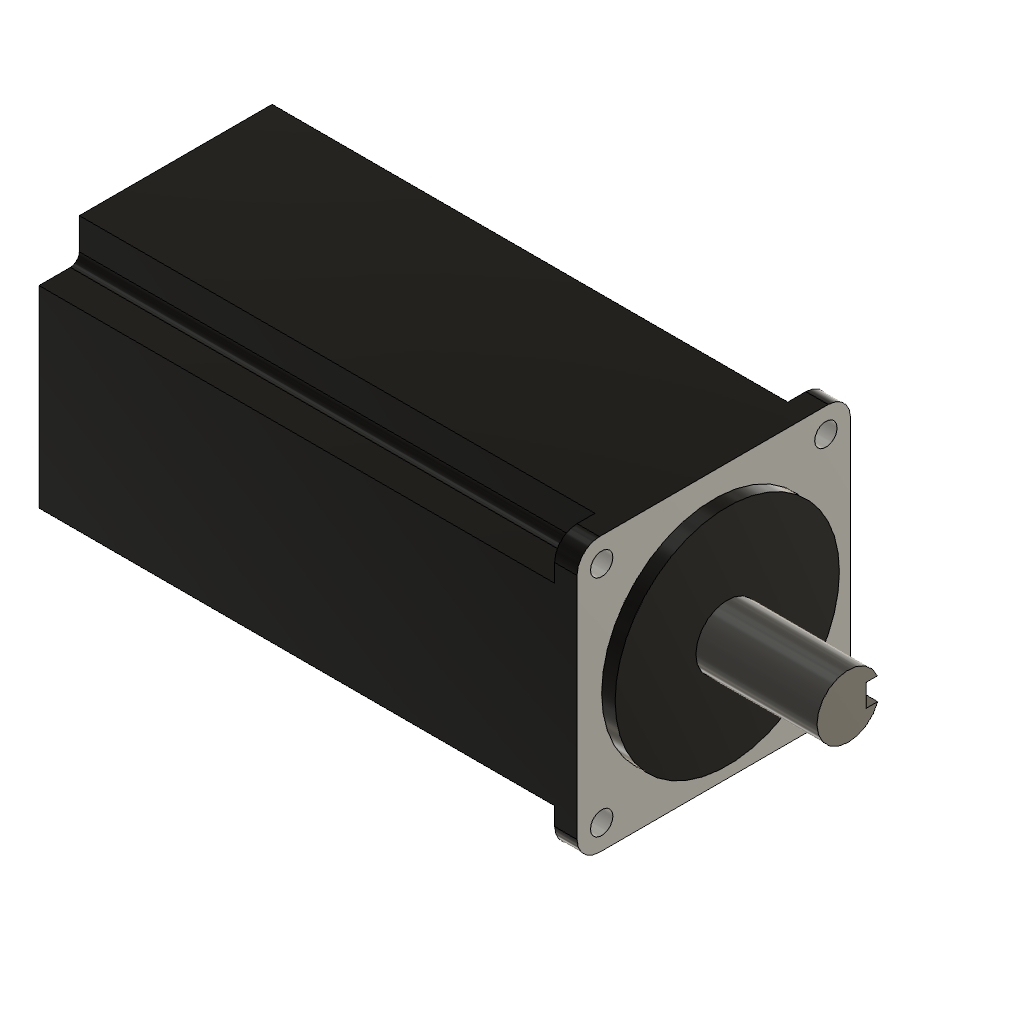
RobotRKO-dobrane elementy (Autodesk Fusion 360 archive; units mm, degrees)
design "NEMA24 60BL120"
part number: 2026-10-05-21-43-38-421
Autodesk Fusion 360 part; units mm, degrees
note: some values were not read from the file. Chosen so that the rebuilt part matches the saved one: a direction. Set by a fixed rule: which sketch regions a step uses.
sketch "Szkic1" plane through (0, 0, 0) normal (1, 0, 0) x (0, 1, 0)
  line L0 (30.5, 30.5) -> (-30.5, 30.5)
  line L1 (-30.5, 30.5) -> (-30.5, -30.5)
  line L2 (-30.5, -30.5) -> (30.5, -30.5)
  line L3 (30.5, -30.5) -> (30.5, 30.5)
  line L4 (30.5, 30.5) -> (-30.5, -30.5) construction
  line L5 (-30.5, 30.5) -> (30.5, -30.5) construction
  dimension "d1" = 61
  dimension "d2" = 61
  constraint horizontal L0
  constraint perpendicular L0 L1
  constraint parallel L0 L2
  constraint parallel L1 L3
  constraint coincident L4 origin
  constraint coincident L5 origin
  measures "d1" distance of L0.start L2.end
  measures "d2" distance of L1.end L2.end
extrude "Wyciągnięcie proste1" add sketch "Szkic1" along normal blind 120
sketch "Szkic2" plane through (120, 0, 0) normal (1, 0, 0) x (0, 1, 0)
  line L0 (30.5, -30.5) -> (30.5, 30.5)
  line L1 (30.5, 30.5) -> (-30.5, 30.5)
  line L2 (-30.5, 30.5) -> (-30.5, -30.5)
  line L3 (-30.5, -30.5) -> (30.5, -30.5)
  circle A0 centre (0, 0) radius 25
  dimension "d5" = 50
  constraint coincident A0.centre origin
  measures "d5" diameter of A0
extrude "Wyciągnięcie proste2" add sketch "Szkic2" along normal blind 3 contours A0
sketch "Szkic3" plane through (123, 0, 0) normal (1, 0, 0) x (0, 1, 0)
  circle A0 centre (0, 0) radius 25
  circle A1 centre (0, 0) radius 7
  dimension "d8" = 14
  constraint concentric A0 A1
  measures "d8" diameter of A1
extrude "Wyciągnięcie proste3" add sketch "Szkic3" along normal blind 27 contours A1
sketch "Szkic4" plane through (150, 0, 0) normal (1, 0, 0) x (0, 1, 0)
  circle A0 centre (0, 0) radius 7
  line L0 (4, -2.4) -> (4, 2.6)
  line L1 (4, 2.6) -> (6.4992, 2.6)
  line L2 (4, -2.4) -> (6.5757, -2.4)
  point P0 (4, 0.1)
  dimension "d11" = 5
  dimension "d12" = 4
  constraint midpoint L0 P0
  constraint vertical L0
  constraint coincident A0 L1.end
  constraint perpendicular L0 L1
  constraint coincident A0 L2.end
  constraint perpendicular L0 L2
  measures "d11" distance of L0.start L0.end
  measures "d12" distance of A0.centre L0
extrude "Wyciągnięcie proste4" cut sketch "Szkic4" against normal blind 25 contours A0 L0 L1 L2 picked at (5, 0.0667)
sketch "Szkic6" plane through (120, 0, 0) normal (1, 0, 0) x (0, 1, 0)
  circle A0 centre (0, 0) radius 25
  line L0 (30.5, -30.5) -> (30.5, 30.5)
  line L1 (30.5, 30.5) -> (-30.5, 30.5)
  line L2 (-30.5, 30.5) -> (-30.5, -30.5)
  line L3 (-30.5, -30.5) -> (30.5, -30.5)
  line L4 (25, -25) -> (-25, -25) construction
  line L5 (-25, -25) -> (-25, 25) construction
  line L6 (-25, 25) -> (25, 25) construction
  line L7 (25, 25) -> (25, -25) construction
  line L8 (25, -25) -> (-25, 25) construction
  line L9 (-25, -25) -> (25, 25) construction
  circle A1 centre (-25, 25) radius 2.5
  circle A2 centre (25, 25) radius 2.5
  circle A3 centre (-25, -25) radius 2.5
  circle A4 centre (25, -25) radius 2.5
  dimension "d15" = 50
  dimension "d16" = 50
  dimension "d17" = 5
  dimension "d20" = 50
  dimension "d21" = -50
  constraint horizontal L4
  constraint perpendicular L4 L5
  constraint parallel L4 L6
  constraint parallel L5 L7
  constraint coincident L8 A0.centre
  constraint coincident L9 A0.centre
  constraint coincident A0.centre origin
  constraint coincident L5.end L6.start
  measures "d15" distance of L4.start L6.end
  measures "d16" distance of L5.end L6.end
  measures "d17" diameter of A1
extrude "Wyciągnięcie proste5" cut sketch "Szkic6" against normal blind 120 contours A1 | A2 | A3 | A4
ref_plane "Płaszczyzna konstrukcyjna1" through (110, 0, 0) normal (1, 0, 0) x (0, 0, -1)
sketch "Szkic7" plane through (110, 0, 0) normal (1, 0, 0) x (0, 1, 0)
  line L0 (30.5, 30.5) -> (21.5, 30.5)
  line L1 (21.5, 30.5) -> (21.5, 23.5)
  line L2 (23.5, 21.5) -> (30.5, 21.5)
  line L3 (30.5, 21.5) -> (30.5, 30.5)
  arc A0 (21.5, 23.5) -> (23.5, 21.5) centre (23.5, 23.5) ccw
  line L4 (-30.5, 30.5) -> (-21.5, 30.5)
  line L5 (-21.5, 30.5) -> (-21.5, 23.5)
  line L6 (-23.5, 21.5) -> (-30.5, 21.5)
  line L7 (-30.5, 21.5) -> (-30.5, 30.5)
  arc A1 (-23.5, 21.5) -> (-21.5, 23.5) centre (-23.5, 23.5) ccw
  line L8 (-30.5, -30.5) -> (-21.5, -30.5)
  line L9 (-21.5, -30.5) -> (-21.5, -23.5)
  line L10 (-23.5, -21.5) -> (-30.5, -21.5)
  line L11 (-30.5, -21.5) -> (-30.5, -30.5)
  arc A2 (-21.5, -23.5) -> (-23.5, -21.5) centre (-23.5, -23.5) ccw
  line L12 (30.5, -30.5) -> (21.5, -30.5)
  line L13 (21.5, -30.5) -> (21.5, -23.5)
  line L14 (23.5, -21.5) -> (30.5, -21.5)
  line L15 (30.5, -21.5) -> (30.5, -30.5)
  arc A3 (23.5, -21.5) -> (21.5, -23.5) centre (23.5, -23.5) ccw
  dimension "d29" = 9
  dimension "d30" = 9
  dimension "d31" = 2
  dimension "d32" = 9
  dimension "d33" = 9
  dimension "d34" = 2
  dimension "d35" = 9
  dimension "d36" = 9
  dimension "d37" = 2
  dimension "d38" = 9
  dimension "d39" = 9
  dimension "d40" = 2
  constraint horizontal L0
  constraint vertical L1
  constraint horizontal L2
  constraint vertical L3
  constraint tangent L1 A0
  constraint tangent L2 A0
  constraint horizontal L4
  constraint vertical L5
  constraint horizontal L6
  constraint vertical L7
  constraint tangent L5 A1
  constraint tangent L6 A1
  constraint horizontal L8
  constraint vertical L9
  constraint horizontal L10
  constraint vertical L11
  constraint tangent L9 A2
  constraint tangent L10 A2
  constraint horizontal L12
  constraint vertical L13
  constraint horizontal L14
  constraint vertical L15
  constraint tangent L13 A3
  constraint tangent L14 A3
  measures "d29" distance of L0.start L2.end
  measures "d30" distance of L0.start L0.end
  measures "d31" radius of A0
  measures "d32" distance of L4.start L4.end
  measures "d33" distance of L4.start L6.end
  measures "d34" radius of A1
  measures "d35" distance of L8.start L10.end
  measures "d36" distance of L8.start L8.end
  measures "d37" radius of A2
  measures "d38" distance of L12.start L12.end
  measures "d39" distance of L12.start L14.end
  measures "d40" radius of A3
extrude "Wyciągnięcie proste6" cut sketch "Szkic7" along normal blind -110 and the other way blind -5
fillet "Zaokrąglenie1" radius 5 1 edges at (117.5, 30.5, 30.5)
fillet "Zaokrąglenie2" radius 5 1 edges at (117.5, -30.5, 30.5)
fillet "Zaokrąglenie3" radius 5 1 edges at (117.5, -30.5, -30.5)
fillet "Zaokrąglenie4" radius 5 1 edges at (117.5, 30.5, -30.5)

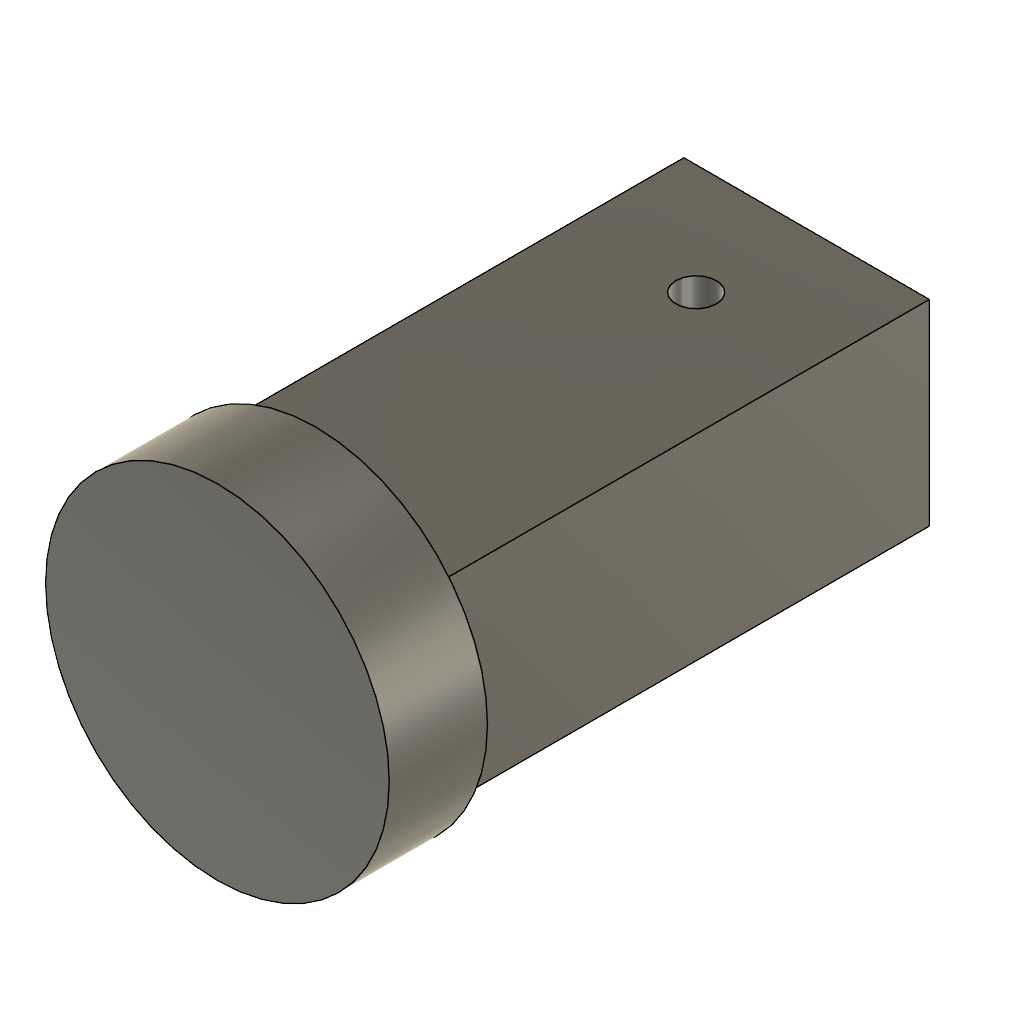
design "pokazowy tlok"
part number: 2026-10-08-21-52-11-483
Autodesk Fusion 360 part; units mm, degrees
sketch "Szkic1" plane through (0, 0, 0) normal (0, 0, 1) x (1, 0, 0)
  line L0 (0, 0) -> (50, 0)
  line L1 (50, 0) -> (50, -100)
  line L2 (50, -100) -> (0, -100)
  line L3 (0, -100) -> (0, 0)
  dimension "d8" = 100
  constraint horizontal L0
  constraint vertical L1
  constraint horizontal L2
  constraint vertical L3
  constraint coincident L0.start L3.end
  measures "d8" distance of L0.end L1.end
extrude "Wyciągnięcie proste1" add sketch "Szkic1" along normal blind 40
sketch "Szkic2" plane through (0, -100, 0) normal (0, -1, 0) x (1, 0, 0)
  line L0 (0, 0) -> (50, 0)
  line L1 (50, 0) -> (50, 40)
  line L2 (50, 40) -> (0, 40)
  line L3 (0, 40) -> (0, 0)
  line L4 (25, 40) -> (25, 0)
  circle A0 centre (25, 20) radius 35
  constraint midpoint L2 L4.start
  constraint midpoint L0 L4.end
  constraint midpoint L4 A0.centre
extrude "Wyciągnięcie proste2" add sketch "Szkic2" along normal blind 20 contours L0 L2 L3 L4 | L0 L1 L2 L4 | A0
sketch "Szkic3" plane through (0, 0, 40) normal (0, 0, 1) x (-1, 0, 0)
  line L0 (0, 100) -> (-50, 100)
  line L1 (-50, 100) -> (-50, 0)
  line L2 (-50, 0) -> (0, 0)
  line L3 (0, 0) -> (0, 100)
  circle A0 centre (-25, 22.5) radius 4.125
  dimension "d5" = 8.25
  dimension "d6" = 22.5
  measures "d5" diameter of A0
  measures "d6" distance of L2 A0.centre
extrude "Wyciągnięcie proste3" cut sketch "Szkic3" against normal through all contours A0

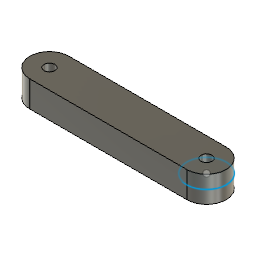
design "korbowodV1RKO"
part number: 2026-08-30-19-32-56-895
Autodesk Fusion 360 part; units mm, degrees
sketch "Szkic1" plane through (0, 0, 0) normal (0, 0, 1) x (1, 0, 0)
  line L0 (60, -15) -> (-60, -15)
  line L1 (-60, 15) -> (60, 15)
  line L2 (60, 4.125) -> (60, -4.125)
  line L3 (60, -15) -> (-60, 15) construction
  line L4 (-60, -15) -> (60, 15) construction
  circle A0 centre (-60, 0) radius 4.125
  circle A1 centre (-60, 0) radius 15
  circle A2 centre (60, 0) radius 4.125
  circle A3 centre (60, 0) radius 15
  dimension "d1" = 30
  dimension "d2" = 120
  dimension "d3" = 8.25
  dimension "d4" = 8.25
  constraint horizontal L0
  constraint parallel L0 L1
  constraint coincident L3 origin
  constraint coincident L4 origin
  constraint concentric A0 A1
  constraint coincident L0.end A1
  constraint concentric A2 A3
  constraint coincident L0.start A3
  constraint coincident A2 L2.end
  constraint coincident L2 A2.centre
  constraint coincident A2 L2.start
  measures "d1" distance of L0.start L1.end
  measures "d2" distance of L1.start L1.end
  measures "d3" diameter of A0
  measures "d4" diameter of A2
extrude "Wyciągnięcie proste1" add sketch "Szkic1" along normal blind 20
ref_plane "Płaszczyzna konstrukcyjna1" through (0, 0, 10) normal (0, 0, 1) x (1, 0, 0)
sketch "Szkic2" plane through (0, 0, 10) normal (0, 0, 1) x (1, 0, 0)
ref_plane "Płaszczyzna konstrukcyjna2" through (0, 0, 10) normal (0, 0, 1) x (1, 0, 0)
sketch "Szkic3" plane through (0, 0, 10) normal (0, 0, 1) x (1, 0, 0)
  circle A0 centre (60, 0) radius 15
  dimension "d12" = 30
  measures "d12" diameter of A0

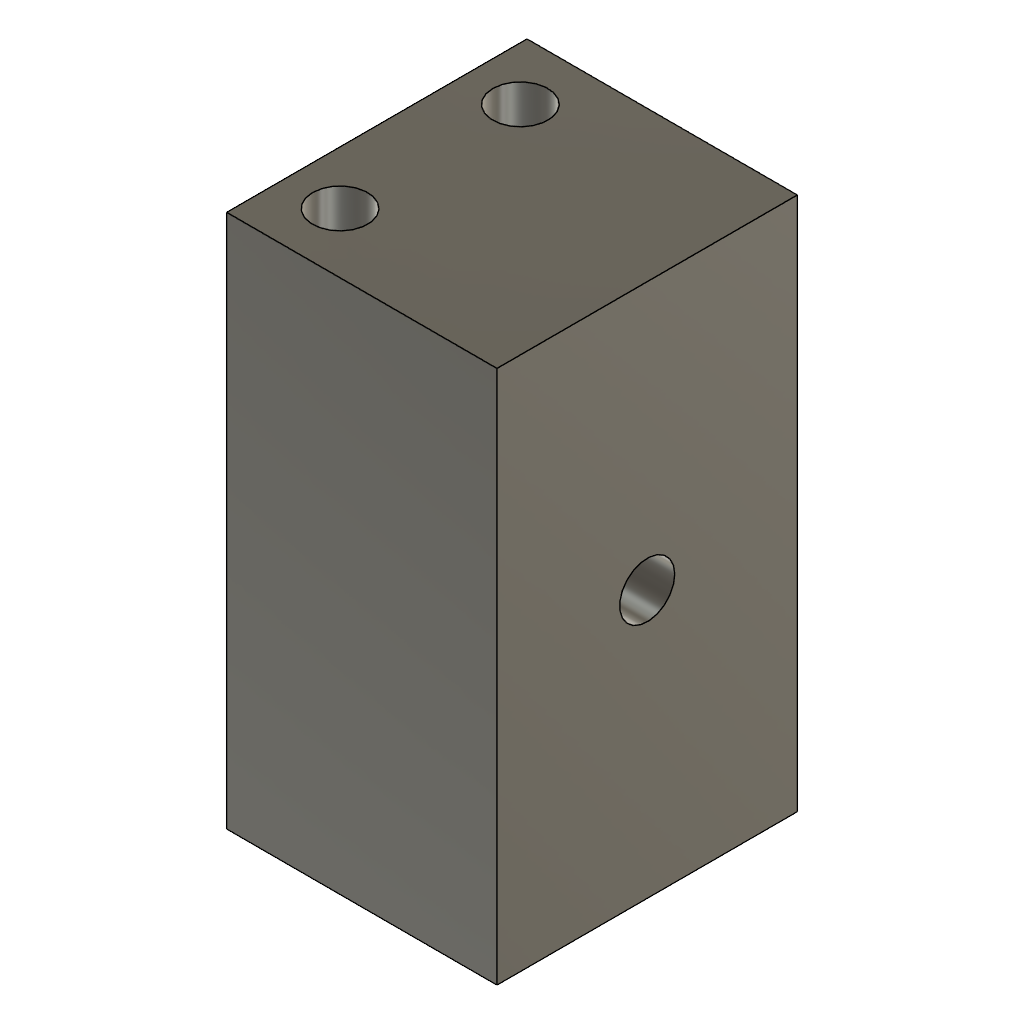
design "suwak"
description: STEP AP214
part number: 2026_10_08_13_11_08_0056
Autodesk Fusion 360 part; units mm, degrees
ref_plane "Płaszczyzna konstrukcyjna1" through (-4.75, 22.5, 25.8) normal (0, 0, 1) x (1, 0, 0)
sketch "Szkic1" plane through (0, 0, 25.8) normal (0, 0, 1) x (1, 0, 0)
  line L0 (-25, 45) -> (15.5, 45)
  line L1 (15.5, 45) -> (15.5, 0)
  line L2 (15.5, 0) -> (-25, 0)
  line L3 (-25, 0) -> (-25, 45)
  circle A0 centre (-17, 36) radius 4.1231
  circle A1 centre (-17, 9) radius 4.1231
  dimension "d5" = 0
  dimension "d6" = -27
  dimension "d9" = 45
  constraint horizontal L0
  constraint vertical L1
  constraint horizontal L2
  constraint vertical L3
  measures "d9" distance of L0.end L1.end
extrude "Wyciągnięcie proste1" add sketch "Szkic1" along normal blind 80 contours L0 L1 L2 L3 | A0 | A1
sketch "Szkic2" plane through (-25, 0, 0) normal (-1, 0, 0) x (0, -1, 0)
  line L0 (-45, 25.8) -> (0, 25.8)
  line L1 (0, 25.8) -> (0, 105.8)
  line L2 (0, 105.8) -> (-45, 105.8)
  line L3 (-45, 105.8) -> (-45, 25.8)
  line L4 (-22.5, 25.8) -> (-22.5, 105.8) construction
  constraint midpoint L0 L4.start
  constraint midpoint L2 L4.end
extrude "Wyciągnięcie proste2" cut sketch "Szkic1" along normal blind 90 contours A0 | A1
sketch "Szkic4" plane through (-25, 0, 0) normal (-1, 0, 0) x (0, -1, 0)
  line L0 (-45, 25.8) -> (0, 25.8)
  line L1 (0, 25.8) -> (0, 105.8)
  line L2 (0, 105.8) -> (-45, 105.8)
  line L3 (-45, 105.8) -> (-45, 25.8)
  line L4 (-22.5, 105.8) -> (-22.5, 25.8)
  circle A0 centre (-22.5, 65.8) radius 4.125
  dimension "d15" = 8.25
  constraint midpoint L2 L4.start
  constraint midpoint L0 L4.end
  constraint midpoint L4 A0.centre
  measures "d15" diameter of A0
extrude "Wyciągnięcie proste4" cut sketch "Szkic4" against normal blind 45 contours L4 A0 | L4 A0
